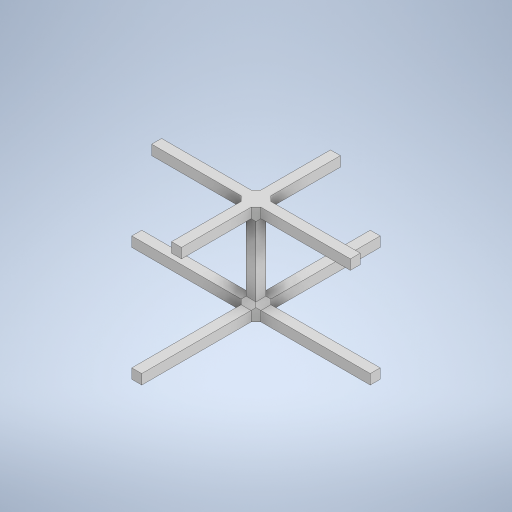
# Autodesk Inventor part: StandSimple
Saved by Autodesk Inventor 2023.4 (Build 274418000, 418)
## iProperties
Created: 2026-02-26
Part Number: StandSimple
Material: Generic
Document SubType Name: Modeling
Designer: 1017208
Density: 1 g/cm^3
Appearance: Default
Author: 1017208
Autodesk Inventor part; units mm, degrees
ref_plane "YZ Plane" through (0, 0, 0) normal (1, 0, 0) x (0, 1, 0)
ref_plane "XZ Plane" through (0, 0, 0) normal (0, 1, 0) x (-1, 0, 0)
ref_plane "XY Plane" through (0, 0, 0) normal (0, 0, 1) x (1, 0, 0)
sketch "Sketch1" plane through (0, 0, 0) normal (0, 1, 0) x (-1, 0, 0)
  line L0 (0, 0) -> (152.4, 0)
  line L1 (76.2, 0) -> (76.2, 76.2)
  line L2 (76.2, 0) -> (152.4, 0) construction
  line L3 (76.2, 0) -> (76.2, -76.2)
  line L4 (76.2, 0) -> (152.4, 0) construction
  line L5 (0, 3.175) -> (152.4, 3.175)
  line L6 (0, -3.175) -> (152.4, -3.175)
  line L7 (152.4, 3.175) -> (152.4, -3.175)
  line L8 (0, 3.175) -> (0, -3.175)
  line L9 (79.375, 76.2) -> (79.375, 0)
  line L10 (79.375, 0) -> (79.375, -76.2)
  line L11 (73.025, 76.2) -> (73.025, 0)
  line L12 (73.025, 0) -> (73.025, -76.2)
  line L13 (79.375, 76.2) -> (73.025, 76.2)
  line L14 (79.375, -76.2) -> (73.025, -76.2)
  point P0 (73.025, 3.175)
  point P1 (73.025, -3.175)
  point P2 (79.375, -3.175)
  point P3 (79.375, 3.175)
  dimension "d0" = 152.4
  dimension "d1" = 76.2
  dimension "d2" = 90
  dimension "d3" = 76.2
  dimension "d4" = 90
  dimension "d5" = 3.175
  dimension "d6" = 3.175
  dimension "d7" = 3.175
  dimension "d8" = 3.175
  constraints: 30 end point, 5 horizontal, 4 vertical, 2 parallel, 2 perpendicular, 1 midpoint, 2 other
  measures "d0" distance of L0.start L0.end
  measures "d1" distance of L1.start L1.end
  measures "d2" angle of L2 L1
  measures "d3" distance of L1.start L3.end
  measures "d4" angle of L3 L4
  measures "d5" distance between parallel lines of L0 L5
  measures "d6" distance between parallel lines of L0 L6
  measures "d7" distance between parallel lines of L1 L9
  measures "d8" distance between parallel lines of L1 L11
extrude "Extrusion1" add sketch "Sketch1" along normal blind 6.35
sketch "Sketch2" plane through (0, 6.35, 0) normal (0, 1, 0) x (1, 0, 0)
  line L0 (-73.025, -3.175) -> (0, -3.175) projected
  line L1 (-79.375, 3.175) -> (-73.025, 3.175)
  line L2 (-73.025, 3.175) -> (-73.025, -3.175)
  line L3 (-73.025, -3.175) -> (-79.375, -3.175)
  line L4 (-79.375, -3.175) -> (-79.375, 3.175)
  point P0 (0, 0)
  constraints: 8 end point, 2 parallel, 1 horizontal, 1 perpendicular
extrude "Extrusion2" add sketch "Sketch2" along normal blind 50.8
sketch "Sketch3" plane through (0, 57.15, 0) normal (0, 1, 0) x (1, 0, 0)
  line L0 (-76.2, 0) -> (-76.2, 50.8)
  line L1 (-76.2, 0) -> (-76.2, -50.8)
  line L2 (-76.2, 0) -> (-12.7, 0)
  line L3 (-76.2, 0) -> (-139.7, 0)
  line L4 (-73.025, 0) -> (-73.025, 50.8)
  line L5 (-73.025, 0) -> (-73.025, -50.8)
  line L6 (-79.375, 0) -> (-79.375, 50.8)
  line L7 (-79.375, 0) -> (-79.375, -50.8)
  line L8 (-76.2, 3.175) -> (-12.7, 3.175)
  line L9 (-76.2, -3.175) -> (-12.7, -3.175)
  line L10 (-76.2, 3.175) -> (-139.7, 3.175)
  line L11 (-76.2, -3.175) -> (-139.7, -3.175)
  line L12 (-79.375, 50.8) -> (-73.025, 50.8)
  line L13 (-139.7, 3.175) -> (-139.7, -3.175)
  line L14 (-73.025, -50.8) -> (-79.375, -50.8)
  line L15 (-73.025, -76.2) -> (-73.025, -3.175) projected
  line L16 (-12.7, 3.175) -> (-12.7, -3.175)
  line L17 (0, 3.175) -> (-73.025, 3.175) projected
  point P0 (0, 0)
  point P1 (-79.375, -3.175)
  point P2 (-73.025, -3.175)
  point P3 (-73.025, 3.175)
  point P4 (-79.375, 3.175)
  dimension "d13" = 50.8
  dimension "d14" = 50.8
  dimension "d15" = 63.5
  dimension "d16" = 63.5
  dimension "d17" = 3.175
  dimension "d18" = 3.175
  dimension "d19" = 3.175
  dimension "d20" = 3.175
  dimension "d21" = 3.175
  dimension "d22" = 3.175
  dimension "d23" = 3.175
  dimension "d24" = 3.175
  constraints: 32 end point, 8 parallel, 3 horizontal, 3 perpendicular, 2 vertical
  measures "d13" distance of L0.start L0.end
  measures "d14" distance of L0.start L1.end
  measures "d15" distance of L0.start L2.end
  measures "d16" distance of L0.start L3.end
  measures "d17" distance between parallel lines of L0 L4
  measures "d18" distance between parallel lines of L1 L5
  measures "d19" distance between parallel lines of L0 L6
  measures "d20" distance between parallel lines of L1 L7
  measures "d21" distance between parallel lines of L2 L8
  measures "d22" distance between parallel lines of L2 L9
  measures "d23" distance between parallel lines of L3 L10
  measures "d24" distance between parallel lines of L3 L11
extrude "Extrusion3" add sketch "Sketch3" along normal blind 6.35
chamfer "Chamfer1" distance 3.175 angle 45 4 edges at (-76.2, 6.35, 3.175) (-73.025, 6.35, 0) (-76.2, 6.35, -3.175) (-79.375, 6.35, 0)
chamfer "Chamfer2" distance 3.175 angle 45 4 edges at (-76.2, 57.15, -3.175) (-79.375, 57.15, 0) (-76.2, 57.15, 3.175) (-73.025, 57.15, 0)
chamfer "Chamfer3" distance 3.175 angle 45 8 edges at (-73.025, 4.7625, 3.175) (-73.025, 58.7375, 3.175) (-73.025, 58.7375, -3.175) (-73.025, 4.7625, -3.175) (-79.375, 58.7375, -3.175) (-79.375, 4.7625, -3.175) (-79.375, 58.7375, 3.175) (-79.375, 4.7625, 3.175)
body "Solid1"
